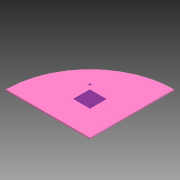
# Autodesk Inventor part: carrier-wafer
Saved by Autodesk Inventor 2011 SP1 (Build 150282100, 282)
## iProperties
Created: 2011-03-23
Part Number: carrier-wafer
Document SubType Name: Modeling
Designer: Andrew Zonenberg
Density: 1 g/cm^3
Author: Andrew Zonenberg
Autodesk Inventor part; units mm, degrees
ref_plane "YZ Plane" through (0, 0, 0) normal (1, 0, 0) x (0, 1, 0)
ref_plane "XZ Plane" through (0, 0, 0) normal (0, 1, 0) x (-1, 0, 0)
ref_plane "XY Plane" through (0, 0, 0) normal (0, 0, 1) x (1, 0, 0)
sketch "Sketch1" plane through (0, 0, 0) normal (0, 0, 1) x (1, 0, 0)
  line L0 (0, 0) -> (-50, 0)
  line L1 (0, 0) -> (0, 50)
  arc A0 (0, 50) -> (-50, 0) centre (0, 0) ccw
  dimension "d0" = 50
  constraints: 4 end point, 2 perpendicular, 2 point on circle, 1 centre point, 1 coincident, 1 horizontal
  measures "d0" distance of L0.start L0.end
extrude "Wafer" add sketch "Sketch1" along normal blind 0.525
fillet "OutsideEdge" radius 0.1 1 edges at (-35.3553, 35.3553, 0.525)
sketch "Sketch3" plane through (0, 0, 0) normal (0, 0, -1) x (-1, 0, 0)
  line L0 (0, 50) -> (0, 0)
  arc A0 (49.9, 0) -> (0, 49.9) centre (0, 0) ccw projected
  line L1 (0, 0) -> (49.9, 0) projected
  line L2 (0, 49.9) -> (0, 0) projected
  constraints: 2 end point
extrude "Wax" add sketch "Sketch3" along normal blind 0.25
sketch "Sketch4" plane through (0, 0, 0.525) normal (0, 0, 1) x (1, 0, 0)
  line L0 (0, 0) -> (-49.9, 0) projected
  line L1 (0, 49.9) -> (0, 0) projected
  line L2 (-24.5, 24.5) -> (-15.5, 24.5) construction
  line L3 (-15.5, 24.5) -> (-15.5, 15.5) construction
  line L4 (-15.5, 15.5) -> (-24.5, 15.5) construction
  line L5 (-24.5, 15.5) -> (-24.5, 24.5) construction
  line L6 (-24.5, 20) -> (-15.5, 20) construction
  line L7 (-20, 24.5) -> (-20, 15.5) construction
  line L8 (-25, 25) -> (-15, 25)
  line L9 (-15, 25) -> (-15, 15)
  line L10 (-15, 15) -> (-25, 15)
  line L11 (-25, 15) -> (-25, 25)
  line L12 (-20, 25) -> (-20, 24.5) construction
  line L13 (-15, 20) -> (-15.5, 20) construction
  line L14 (-27.75, 27.75) -> (-27.25, 27.75) construction
  line L15 (-27.25, 27.75) -> (-27.25, 27.25) construction
  line L16 (-27.25, 27.25) -> (-27.75, 27.25) construction
  line L17 (-27.75, 27.25) -> (-27.75, 27.75) construction
  line L18 (-27.75, 27.5) -> (-27.25, 27.5) construction
  line L19 (-27.5, 27.75) -> (-27.5, 27.25) construction
  line L20 (-27.75, 27.75) -> (-27.75, 28.25)
  line L21 (-27.75, 28.25) -> (-27.25, 28.25)
  line L22 (-27.25, 28.25) -> (-27.25, 27.75)
  line L23 (-27.25, 27.75) -> (-26.75, 27.75)
  line L24 (-26.75, 27.75) -> (-26.75, 27.25)
  line L25 (-26.75, 27.25) -> (-27.25, 27.25)
  line L26 (-27.25, 27.25) -> (-27.25, 26.75)
  line L27 (-27.25, 26.75) -> (-27.75, 26.75)
  line L28 (-27.75, 26.75) -> (-27.75, 27.25)
  line L29 (-27.75, 27.25) -> (-28.25, 27.25)
  line L30 (-28.25, 27.25) -> (-28.25, 27.75)
  line L31 (-28.25, 27.75) -> (-27.75, 27.75)
  point P0 (-20, 20)
  point P1 (-20, 20)
  point P2 (-20, 20)
  dimension "d8" = 20
  dimension "d9" = 20
  dimension "d10" = 9
  dimension "d11" = 10
  dimension "d14" = 0.5
  dimension "d15" = 2.5
  dimension "d16" = 2.5
  constraints: 60 end point, 11 midpoint, 11 parallel, 11 perpendicular, 8 equal length, 4 horizontal, 2 coincident
  measures "d8" distance from line of L1 point (-20, 20)
  measures "d9" distance from line of L0 point (-20, 20)
  measures "d10" distance of L2.start L2.end
  measures "d11" distance between parallel lines of L9 L11
  measures "d14" distance between parallel lines of L15 L17
  measures "d15" distance between parallel lines of L11 L19
  measures "d16" distance between parallel lines of L8 L18
extrude "Cutout" cut sketch "Sketch4" against normal blind 0.1 draft -57.6
body "Solid1"
